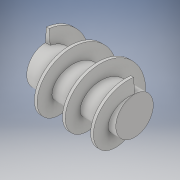
# Autodesk Inventor part: rollers
Saved by Autodesk Inventor 2019 (Build 230136000, 136)
## iProperties
Created: 2020-02-19
Part Number: rollers
Material: Generic
Document SubType Name: Modeling
Designer: ACHYUTH
Density: 1 g/cm^3
Appearance: Default
Author: ACHYUTH
Autodesk Inventor part; units mm, degrees
ref_plane "YZ Plane" through (0, 0, 0) normal (1, 0, 0) x (0, 1, 0)
ref_plane "XZ Plane" through (0, 0, 0) normal (0, 1, 0) x (-1, 0, 0)
ref_plane "XY Plane" through (0, 0, 0) normal (0, 0, 1) x (1, 0, 0)
sketch "Sketch1" plane through (0, 0, 0) normal (0, 0, 1) x (1, 0, 0)
  line L0 (0, 20) -> (5, 20)
  line L1 (4, 35) -> (5, 20)
  line L2 (1, 35) -> (0, 20)
  line L3 (1, 35) -> (4, 35)
  point P0 (0, 0)
  dimension "d1" = 5
  constraints: 8 end point, 2 horizontal
  measures "d1" distance of L0.start L0.end
coil "Coil1" sketch "Sketch1" operation add axis through (-10, 0, 0) along (1, 0, 0) pitch 30 turns 3 hand left
sketch "Sketch2" plane through (0, 0, 0) normal (1, 0, 0) x (0, 1, 0)
  circle A0 centre (0, 0) radius 20
  point P0 (20, 0)
  constraints: 1 coincident, 1 horizontal alignment, 2 other
extrude "Extrusion1" add sketch "Sketch2" along normal blind 95
body "Solid1"
